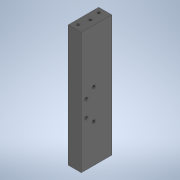
# Autodesk Inventor part: thigh2x4
Saved by Autodesk Inventor 2021.5 (Build 255421000, 421)
## iProperties
Created: 2024-11-18
Part Number: thigh2x4
Material: Wood (Birch)
Document SubType Name: Modeling
Designer: email
Density: 0.55 g/cm^3
Appearance: Birch - Natural Polished
Author: email
Autodesk Inventor part; units mm, degrees
ref_plane "YZ Plane" through (0, 0, 0) normal (1, 0, 0) x (0, 1, 0)
ref_plane "XZ Plane" through (0, 0, 0) normal (0, 1, 0) x (-1, 0, 0)
ref_plane "XY Plane" through (0, 0, 0) normal (0, 0, 1) x (1, 0, 0)
sketch "Sketch1" plane through (0, 0, 0) normal (0, 1, 0) x (-1, 0, 0)
  line L0 (0, 0) -> (-38.1, 0)
  line L1 (-38.1, 0) -> (-38.1, -88.9)
  line L2 (-38.1, -88.9) -> (0, -88.9)
  line L3 (0, -88.9) -> (0, 0)
  dimension "d0" = 38.1
  dimension "d1" = 88.9
  constraints: 8 end point, 2 parallel, 1 horizontal, 1 perpendicular
  measures "d0" distance of L1.end L2.end
  measures "d1" distance of L0.end L1.end
extrude "Extrusion1" add sketch "Sketch1" along normal blind 355.6
sketch "Sketch3" plane through (0, 355.6, 0) normal (0, 1, 0) x (1, 0, 0)
  line L0 (14.2, 74.725) -> (14.2, 14.175)
  line L1 (38.1, 88.9) -> (0, 88.9) projected
  line L2 (0, 0) -> (38.1, 0) projected
  line L3 (14.2, 44.45) -> (20.2, 44.45)
  line L4 (0, 88.9) -> (0, 0) projected
  dimension "d59" = 60.55
  dimension "d60" = 14.175
  dimension "d61" = 14.175
  dimension "d62" = 6
  dimension "d63" = 30.275
  dimension "d64" = 20.2
  constraints: 4 end point, 1 horizontal, 1 midpoint, 1 vertical
  measures "d59" distance of L0.start L0.end
  measures "d60" distance from line of L1 L0.start
  measures "d61" distance from line of L2 L0.end
  measures "d62" distance of L3.start L3.end
  measures "d63" distance from line of L0.start L3
  measures "d64" distance from line of L4 L3.end
hole "Hole1" at (14.2, 355.6, -74.725) at (20.2, 355.6, -44.45) at (14.2, 355.6, -14.175) direction (0, -1, 0) diameter 7 depth 10 tip angle 118
sketch "Sketch5" plane through (38.1, 0, -88.9) normal (0, 0, -1) x (-1, 0, 0)
  line L0 (0, 355.6) -> (28.2843, 327.3157)
  line L1 (0, 355.6) -> (38.1, 355.6) projected
  circle A0 centre (28.2843, 327.3157) radius 2.35
  circle A1 centre (15.5563, 340.0437) radius 2.35
  point P0 (38.1, 0)
  dimension "d25" = 45
  dimension "d26" = 40
  dimension "d27" = 4.7
  dimension "d28" = 4.7
  dimension "d29" = 18
  constraints: 2 centre point, 2 end point, 1 coincident, 1 point on line
  measures "d25" angle of L1 L0
  measures "d26" distance of L0.start L0.end
  measures "d27" diameter of A1
  measures "d28" diameter of A0
  measures "d29" distance of A1.centre L0.end
hole "Hole2" at (9.8157, 327.3157, -88.9) at (22.5437, 340.0437, -88.9) direction (0, 0, 1) diameter 6.5 depth 10
sketch "Sketch6" plane through (38.1, 0, -88.9) normal (0, 0, -1) x (-1, 0, 0)
  line L0 (0, 0) -> (0, 355.6) projected
  line L1 (0, 0) -> (30, 0)
  line L2 (30, 0) -> (30, 20)
  line L3 (30, 20) -> (0, 20)
  line L4 (0, 20) -> (0, 0)
  line L5 (30, 20) -> (30, 68.9)
  circle A0 centre (30, 20) radius 6.1957
  circle A1 centre (30, 68.9) radius 5.1366
  point P0 (38.1, 0)
  dimension "d37" = 30
  dimension "d38" = 20
  dimension "d39" = 48.9
  constraints: 10 end point, 2 centre point, 2 coincident, 2 parallel, 1 horizontal, 1 perpendicular, 1 vertical
  measures "d37" distance of L2.end L3.end
  measures "d38" distance of L1.end L2.end
  measures "d39" distance of L2.end L5.end
hole "Hole3" at (8.1, 20, -88.9) at (8.1, 68.9, -88.9) direction (0, 0, 1) diameter 6.5 depth 10
sketch "Sketch7" plane through (38.1, 0, 0) normal (1, 0, 0) x (0, 0, -1)
  line L0 (0, 0) -> (36, 0)
  line L1 (36, 0) -> (36, 200)
  line L2 (36, 200) -> (0, 200)
  line L3 (0, 200) -> (0, 0)
  circle A0 centre (36, 200) radius 3.75
  circle A1 centre (36, 112.15) radius 3.75
  dimension "d47" = 36
  dimension "d48" = 200
  dimension "d49" = 87.85
  dimension "d50" = 7.5
  dimension "d51" = 7.5
  dimension "d65" = 112.15
  constraints: 8 end point, 2 centre point, 2 parallel, 1 coincident, 1 horizontal, 1 perpendicular, 1 point on line
  measures "d47" distance of L1.end L2.end
  measures "d48" distance of L0.end L1.end
  measures "d49" distance of L1.end A1.centre
  measures "d50" diameter of A1
  measures "d51" diameter of A0
  measures "d65" distance from line of L0 A1.centre
hole "Hole4" at (38.1, 112.15, -36) at (38.1, 200, -36) direction (-1, 0, 0) diameter 7.5 depth 10
sketch "Sketch8" plane through (38.1, 0, 0) normal (1, 0, 0) x (0, 0, -1)
  line L0 (0, 0) -> (14, 0)
  line L1 (14, 0) -> (14, 156.083) construction
  line L2 (14, 156.083) -> (0, 156.083)
  line L3 (0, 156.083) -> (0, 0)
  line L4 (14, 156.083) -> (14, 132.083)
  line L5 (14, 156.083) -> (14, 180.083)
  circle A0 centre (14, 132.083) radius 4
  circle A1 centre (14, 180.083) radius 4
  dimension "d66" = 156.083
  dimension "d67" = 14
  dimension "d69" = 24
  dimension "d70" = 24
  dimension "d71" = 8
  dimension "d72" = 8
  constraints: 12 end point, 2 centre point, 2 coincident, 2 parallel, 1 horizontal, 1 perpendicular, 1 point on line, 1 vertical
  measures "d66" distance of L0.end L1.end
  measures "d67" distance of L1.end L2.end
  measures "d69" distance of L1.end L4.end
  measures "d70" distance of L5.end L1.end
  measures "d71" diameter of A0
  measures "d72" diameter of A1
extrude "Extrusion2" cut sketch "Sketch8" against normal blind 10
body "Solid1"
